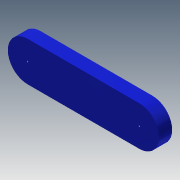
# Autodesk Inventor part: tahlo5(b)_sablona
Saved by Autodesk Inventor 2013 (Build 170138000, 138)
## iProperties
Created: 2013-02-02
Part Number: tahlo5(b)_sablona
Material: Generic
Document SubType Name: Modeling
Designer: idle-rug
Density: 1 g/cm^3
Author: idle-rug
Autodesk Inventor part; units mm, degrees
ref_plane "YZ Plane" through (0, 0, 0) normal (1, 0, 0) x (0, 1, 0)
ref_plane "XZ Plane" through (0, 0, 0) normal (0, 1, 0) x (-1, 0, 0)
ref_plane "XY Plane" through (0, 0, 0) normal (0, 0, 1) x (1, 0, 0)
sketch "Sketch1" plane through (0, 0, 0) normal (0, 1, 0) x (-1, 0, 0)
  line L0 (-8.5, -3) -> (8.5, -3)
  line L1 (8.5, -3) -> (8.5, 3)
  line L2 (8.5, 3) -> (-8.5, 3)
  line L3 (-8.5, 3) -> (-8.5, -3)
  line L4 (-8.5, -3) -> (8.5, 3) construction
  line L5 (8.5, -3) -> (-8.5, 3) construction
  circle A0 centre (8.5, 0) radius 3
  circle A1 centre (-8.5, 0) radius 3
  point P0 (0, 0)
  dimension "d0" = 17
  dimension "d1" = 6
  dimension "d2" = 6
  dimension "d3" = 6
  constraints: 12 end point, 4 midpoint, 2 centre point, 2 parallel, 1 horizontal, 1 perpendicular
  measures "d0" distance of L2.end L1.end
  measures "d1" distance of L1.end L0.end
  measures "d2" diameter of A0
  measures "d3" diameter of A1
extrude "Extrusion1" add sketch "Sketch1" along normal blind 2
sketch "Sketch2" plane through (0, 2, 0) normal (0, 1, 0) x (1, 0, 0)
  arc A0 (8.5, -3) -> (8.5, 3) centre (8.5, 0) ccw projected
  arc A1 (-8.5, 3) -> (-8.5, -3) centre (-8.5, 0) ccw projected
  circle A2 centre (-8.5, 0) radius 1.5
  circle A3 centre (8.5, 0) radius 1.5
  point P0 (0, 0)
  dimension "d6" = 3
  dimension "d7" = 3
  constraints: 2 centre point, 2 coincident
  measures "d6" diameter of A2
  measures "d7" diameter of A3
extrude "Extrusion2" cut sketch "Sketch2" against normal blind 2
sketch "Sketch3" plane through (0, 0, 0) normal (0, -1, 0) x (1, 0, 0)
  circle A0 centre (-8.5, 0) radius 1.5 projected
  circle A1 centre (8.5, 0) radius 1.5 projected
  arc A2 (8.5, -3) -> (8.5, 3) centre (8.5, 0) ccw projected
  arc A3 (-8.5, 3) -> (-8.5, -3) centre (-8.5, 0) ccw projected
  circle A4 centre (-8.5, 0) radius 0.1
  circle A5 centre (8.5, 0) radius 0.1
  point P0 (0, 0)
  dimension "d10" = 0.2
  dimension "d11" = 0.2
  constraints: 2 centre point, 2 coincident
  measures "d10" diameter of A4
  measures "d11" diameter of A5
extrude "Extrusion3" add sketch "Sketch3" against normal blind 2
body "Solid1"
